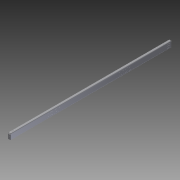
# Autodesk Inventor part: Base Side Bar
Saved by Autodesk Inventor 2012 (Build 160160000, 160)
## iProperties
Created: 2011-10-13
Part Number: Base Side Bar
Material: Default
Document SubType Name: Sheet Metal
Designer: Tushar
Density: 1 g/cm^3
Sheet Metal Rule: Default
Author: Tushar
Autodesk Inventor part; units mm, degrees
ref_plane "YZ Plane" through (0, 0, 0) normal (1, 0, 0) x (0, 1, 0)
ref_plane "XZ Plane" through (0, 0, 0) normal (0, 1, 0) x (-1, 0, 0)
ref_plane "XY Plane" through (0, 0, 0) normal (0, 0, 1) x (1, 0, 0)
sketch "Sketch2" plane through (0, 0, 0) normal (1, 0, 0) x (0, 1, 0)
  line L0 (-22.225, -762) -> (22.225, -762)
  line L1 (22.225, -762) -> (22.225, 762)
  line L2 (22.225, 762) -> (-22.225, 762)
  line L3 (-22.225, 762) -> (-22.225, -762)
  point P0 (0, 0)
  dimension "d0" = 762
  dimension "d1" = 762
  dimension "d2" = 22.225
  dimension "d3" = 22.225
  measures "d0" distance from line of L2 point (0, 0)
  measures "d1" distance from line of L0 point (0, 0)
  measures "d2" distance from line of L1 point (0, 0)
  measures "d3" distance from line of L3 point (0, 0)
extrude "Plate1" add sketch "Sketch2" against normal blind 3.048
sketch "Sketch3" plane through (0, -22.225, 762) normal (0, 0, 1) x (1, 0, 0)
  line L0 (0, 44.45) -> (0, 0)
  arc A0 (0, 44.45) -> (-6.223, 50.673) centre (-6.223, 44.45) ccw
  line L1 (-6.223, 44.45) -> (-6.223, 50.673) construction
  line L2 (-6.223, 44.45) -> (0, 44.45) construction
  line L3 (-6.223, 50.673) -> (-19.5834, 50.673)
  point P0 (0, 22.225)
  point P1 (0, 22.225)
  point P2 (0, 22.225)
  dimension "d5" = 90
  dimension "d7" = 13.3604
  dimension "d11" = 6.223
  measures "d5" angle of L2 L1
  measures "d7" distance of L1.end L3.end
  measures "d11" radius of A0
contour flange "Contour Flange1" sketch "Sketch3" thickness 3.048 bend radius 3.048 curves A0 L3 edges at (0, 22.225, 0) running between points at (0, 22.225, -762) (0, 22.225, 762)
bend "Bend1"
corner "Corner1"
sketch "Sketch4" plane through (-3.048, -22.225, 762) normal (0, 0, 1) x (1, 0, 0)
  line L0 (3.048, 44.45) -> (3.048, 0)
  arc A0 (-3.175, -6.223) -> (3.048, 0) centre (-3.175, 0) ccw
  line L1 (-3.175, 0) -> (-3.175, -6.223) construction
  line L2 (-3.175, 0) -> (3.048, 0) construction
  line L3 (-3.175, -6.223) -> (-16.5354, -6.223)
  point P0 (0, 0)
  point P1 (3.048, 22.225)
  point P2 (3.048, 22.225)
  dimension "d21" = 90
  dimension "d22" = 6.223
  dimension "d23" = 13.3604
  dimension "d24" = 6.223
  measures "d21" angle of L1 L2
  measures "d22" radius of A0
  measures "d23" distance of L1.end L3.end
  measures "d24" vertical distance of point (0, 0) L1.end
contour flange "Contour Flange2" sketch "Sketch4" thickness 3.048 bend radius 3.048 curves L3 A0 edges at (0, -22.225, 0) running between points at (0, -22.225, 762) (0, -22.225, -762)
bend "Bend2"
corner "Corner2"
sketch "Sketch5" plane through (-6.223, 28.448, 762) normal (0, 1, 0) x (1, 0, 0)
  arc A0 (6.223, 1524) -> (0, 1530.223) centre (0, 1524) ccw
  line L0 (0, 1524) -> (0, 1530.223) construction
  line L1 (0, 1524) -> (6.223, 1524) construction
  line L2 (0, 1530.223) -> (-13.3604, 1530.223)
  point P0 (0, 1524)
  point P1 (6.223, 762)
  point P2 (6.223, 1524)
  dimension "d34" = 90
  dimension "d35" = 6.223
  dimension "d36" = 13.3604
  dimension "d37" = 6.223
  measures "d34" angle of L1 L0
  measures "d35" radius of A0
  measures "d36" distance of L0.end L2.end
  measures "d37" distance of point (0, 1524) L0.end
contour flange "Contour Flange3" sketch "Sketch5" thickness 3.048 bend radius 3.048 curves A0 L2 edges at (0, 0, -762) running between points at (0, -22.225, -762) (0, 22.225, -762)
bend "Bend3"
corner "Corner3"
sketch "Sketch6" plane through (-6.223, 28.448, 762) normal (0, 1, 0) x (1, 0, 0)
  arc A0 (0, -6.223) -> (6.223, 0) centre (0, 0) ccw
  line L0 (0, 0) -> (0, -6.223) construction
  line L1 (0, 0) -> (6.223, 0) construction
  line L2 (0, -6.223) -> (-13.3604, -6.223)
  point P0 (0, 0)
  point P1 (6.223, 762)
  point P2 (6.223, 0)
  dimension "d47" = 90
  dimension "d48" = 6.223
  dimension "d49" = 6.223
  dimension "d50" = 13.3604
  measures "d47" angle of L0 L1
  measures "d48" radius of A0
  measures "d49" distance of L0.end point (0, 0)
  measures "d50" distance of L0.end L2.end
contour flange "Contour Flange4" sketch "Sketch6" thickness 3.048 bend radius 3.048 curves L2 A0 edges at (0, 0, 762) running between points at (0, 22.225, 762) (0, -22.225, 762)
bend "Bend4"
corner "Corner4"
sketch "Sketch8" plane through (0, 0, 0) normal (1, 0, 0) x (0, 0, -1)
  line L0 (-762, -22.225) -> (762, -22.225) projected
  line L1 (768.223, 22.225) -> (768.223, -22.225) projected
  point P0 (0, 0)
  point P1 (723.773, -15.748)
  dimension "d60" = 44.45
  dimension "d61" = 6.477
  measures "d60" distance from line of L1 point (723.773, -15.748)
  measures "d61" distance from line of L0 point (723.773, -15.748)
hole "Hole1" at (0, -15.748, -723.773) direction (-1, 0, 0) diameter 3.175 end through all
sketch "Sketch9" plane through (0, 0, 0) normal (1, 0, 0) x (0, 0, -1)
  circle A0 centre (723.773, -15.748) radius 1.5875 projected
  line L0 (-762, -22.225) -> (762, -22.225) projected
  line L1 (723.773, -15.748) -> (749.173, -15.748)
  point P0 (0, 0)
  dimension "d69" = 25.4
  constraints: 2 end point, 1 parallel
  measures "d69" distance of L1.start L1.end
sketch "Sketch10" plane through (0, 0, 0) normal (1, 0, 0) x (0, 0, -1)
  circle A0 centre (723.773, -15.748) radius 1.5875 projected
  line L0 (-762, -22.225) -> (762, -22.225) projected
  line L1 (723.773, -15.748) -> (723.773, 9.652)
  point P0 (0, 0)
  dimension "d70" = 25.4
  constraints: 2 end point, 1 perpendicular
  measures "d70" distance of L1.start L1.end
pattern_linear "Rectangular Pattern1" count 3 spacing 12.7 along (0, 0, -1) count 3 spacing 15.748 along (0, 1, 0) of "Hole1"
sketch "Sketch11" plane through (-6.223, 28.448, 762) normal (0, 1, 0) x (1, 0, 0)
  line L0 (6.223, 1524) -> (6.223, 0) projected
  line L1 (0, 1530.223) -> (-13.3604, 1530.223) projected
  point P0 (6.223, 762)
  point P1 (-9.525, 1455.801)
  point P2 (0, 1455.801)
  point P3 (0, 1465.326)
  point P4 (-9.525, 1465.326)
  dimension "d77" = 15.748
  dimension "d91" = 74.422
  dimension "d92" = 9.525
  dimension "d93" = 9.525
  dimension "d94" = 9.525
  dimension "d95" = 9.525
  constraints: 2 vertical alignment
  measures "d77" distance from line of L0 point (-9.525, 1455.801)
  measures "d91" distance from line of point (-9.525, 1455.801) L1
  measures "d92" distance of point (-9.525, 1455.801) point (0, 1455.801)
  measures "d93" distance of point (-9.525, 1465.326) point (-9.525, 1455.801)
  measures "d94" distance of point (0, 1465.326) point (-9.525, 1465.326)
  measures "d95" distance of point (0, 1455.801) point (0, 1465.326)
hole "Hole3" at (-15.748, 28.448, -693.801) at (-6.223, 28.448, -693.801) at (-6.223, 28.448, -703.326) at (-15.748, 28.448, -703.326) direction (0, -1, 0) diameter 3.175 end through all
sketch "Sketch14" plane through (-6.223, -22.225, -768.223) normal (0, 0, -1) x (-1, 0, 0)
  line L0 (0, -6.223) -> (13.3604, -6.223) projected
  line L1 (-6.223, 0) -> (-6.223, 44.45) projected
  point P0 (-6.223, 22.225)
  point P1 (3.175, 6.477)
  dimension "d103" = 12.7
  dimension "d104" = 9.398
  measures "d103" distance from line of L0 point (3.175, 6.477)
  measures "d104" distance from line of L1 point (3.175, 6.477)
hole "Hole4" at (-9.398, -15.748, -768.223) direction (0, 0, 1) diameter 3.175 end through all
sketch "Sketch15" plane through (-6.223, -22.225, -768.223) normal (0, 0, -1) x (-1, 0, 0)
  circle A0 centre (3.175, 6.477) radius 1.5875 projected
  line L0 (0, 44.45) -> (13.3604, 44.45) projected
  line L1 (3.175, 6.477) -> (3.175, 17.6589)
  point P0 (-6.223, 22.225)
  constraints: 2 end point, 1 perpendicular
pattern_linear "Rectangular Pattern3" count 3 spacing 15.748 along (0, 1, 0) of "Hole4"
sketch "Sketch16" plane through (-3.048, 0, 0) normal (-1, 0, 0) x (0, 0, 1)
  line L0 (762, -25.4) -> (-762, -25.4) projected
  line L1 (-768.223, -22.225) -> (-768.223, 22.225) projected
  line L2 (-762, 25.4) -> (762, 25.4) projected
  line L3 (768.223, 22.225) -> (768.223, -22.225) projected
  point P0 (0, 0)
  point P1 (-374.523, -12.7)
  point P2 (-374.523, 12.7)
  point P3 (298.323, -12.7)
  point P4 (298.323, 12.7)
  dimension "d115" = 12.7
  dimension "d116" = 393.7
  dimension "d117" = 12.7
  dimension "d118" = 393.7
  dimension "d119" = 12.7
  dimension "d120" = 12.7
  dimension "d121" = 469.9
  dimension "d122" = 469.9
  measures "d115" distance from line of L0 point (-374.523, -12.7)
  measures "d116" distance from line of L1 point (-374.523, -12.7)
  measures "d117" distance from line of L2 point (-374.523, 12.7)
  measures "d118" distance from line of L1 point (-374.523, 12.7)
  measures "d119" distance from line of L0 point (298.323, -12.7)
  measures "d120" distance from line of L2 point (298.323, 12.7)
  measures "d121" distance from line of point (298.323, 12.7) L3
  measures "d122" distance from line of point (298.323, -12.7) L3
hole "Hole5" at (-3.048, -12.7, -374.523) at (-3.048, 12.7, -374.523) at (-3.048, -12.7, 298.323) at (-3.048, 12.7, 298.323) direction (1, 0, 0) diameter 3.175 end through all
sketch "Sketch17" plane through (-3.048, 0, 0) normal (-1, 0, 0) x (0, 0, 1)
  circle A0 centre (-374.523, -12.7) radius 1.5875 projected
  line L0 (762, 22.225) -> (762, -22.225) projected
  line L1 (-374.523, -12.7) -> (-352.5869, -12.7)
  point P0 (0, 0)
  constraints: 2 end point, 1 perpendicular
pattern_linear "Rectangular Pattern4" count 9 spacing 12.7 along (0, 0, 1) of "Hole5"
sketch "Sketch18" plane through (-19.5834, 28.448, 762) normal (0, 1, 0) x (1, 0, 0)
  line L0 (13.3604, 0) -> (0, 0) projected
  line L1 (13.3604, 0) -> (13.3604, 1454.2135) projected
  point P0 (19.5834, 762)
  point P1 (8.9154, 21.7424)
  point P2 (4.4704, 28.0924)
  point P3 (8.9154, 34.4424)
  point P4 (4.4704, 40.7924)
  dimension "d133" = 4.445
  dimension "d135" = 21.7424
  dimension "d136" = 6.35
  dimension "d137" = 6.35
  dimension "d138" = 6.35
  dimension "d146" = 4.445
  constraints: 2 vertical alignment
  measures "d133" distance from line of L1 point (8.915, 21.742)
  measures "d135" distance from line of point (8.915, 21.742) L0
  measures "d136" vertical distance of point (4.47, 28.092) point (8.915, 21.742)
  measures "d137" vertical distance of point (8.915, 34.442) point (4.47, 28.092)
  measures "d138" vertical distance of point (8.915, 34.442) point (4.47, 40.792)
  measures "d146" horizontal distance of point (4.47, 28.092) point (8.915, 21.742)
hole "Hole6" at (-10.668, 28.448, 740.2576) at (-15.113, 28.448, 733.9076) at (-10.668, 28.448, 727.5576) at (-15.113, 28.448, 721.2076) direction (0, -1, 0) diameter 3.175 end through all
equation "\"d67\" = Thickness"
equation "\"d101\" = Thickness"
equation "\"d110\" = Thickness"
equation "\"d117\" = d115"
equation "\"d118\" = d116"
equation "\"d119\" = d115"
equation "\"d120\" = d115"
equation "\"d128\" = Thickness"
equation "\"d144\" = Thickness"
equation "\"d12\" = BendReliefWidth"
equation "\"d13\" = BendReliefDepth"
equation "\"d14\" = MinimumRemnant"
equation "\"d15\" = BendRadius"
equation "\"d16\" = BendRadius"
equation "\"d18\" = CornerReliefSize"
equation "\"d19\" = GapSize"
equation "\"d20\" = JacobiRadiusSize"
equation "\"d25\" = BendReliefWidth"
equation "\"d26\" = BendReliefDepth"
equation "\"d27\" = MinimumRemnant"
equation "\"d28\" = BendRadius"
equation "\"d29\" = BendRadius"
equation "\"d31\" = CornerReliefSize"
equation "\"d32\" = GapSize"
equation "\"d33\" = JacobiRadiusSize"
equation "\"d38\" = BendReliefWidth"
equation "\"d39\" = BendReliefDepth"
equation "\"d40\" = MinimumRemnant"
equation "\"d41\" = BendRadius"
equation "\"d42\" = BendRadius"
equation "\"d44\" = CornerReliefSize"
equation "\"d45\" = GapSize"
equation "\"d46\" = JacobiRadiusSize"
equation "\"d51\" = BendReliefWidth"
equation "\"d52\" = BendReliefDepth"
equation "\"d53\" = MinimumRemnant"
equation "\"d54\" = BendRadius"
equation "\"d55\" = BendRadius"
equation "\"d57\" = CornerReliefSize"
equation "\"d58\" = GapSize"
equation "\"d59\" = JacobiRadiusSize"
equation "\"d1\" = d0"
equation "\"d3\" = d2"
equation "\"BendRadius\" = Thickness"
equation "\"BendReliefWidth\" = Thickness"
equation "\"BendReliefDepth\" = 0.5 * Thickness"
equation "\"CornerReliefSize\" = 4 * Thickness"
equation "\"MinimumRemnant\" = 2 * Thickness"
equation "\"TransitionRadius\" = BendRadius"
equation "\"JacobiRadiusSize\" = BendRadius"
equation "\"GapSize\" = Thickness"
equation "\"d4\" = BendRadius"
equation "\"Thickness\" = 3.048"
body "Solid1"
